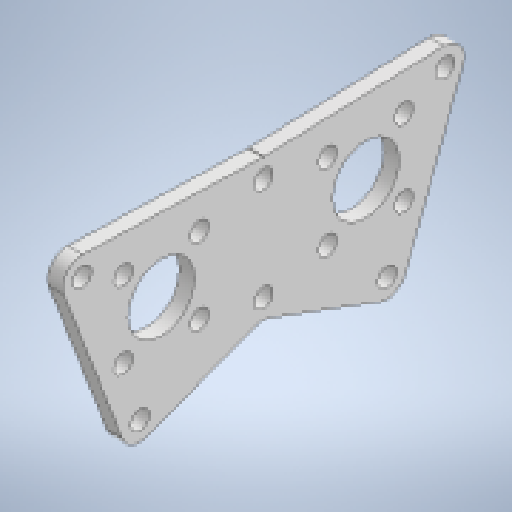
# Autodesk Inventor part: Motor Mount Plate
Saved by Autodesk Inventor 2023 (Build 270158000, 158)
## iProperties
Created: 2022-09-05
Part Number: Motor Mount Plate
Material: Generic
Document SubType Name: Modeling
Designer: deli
Density: 1 g/cm^3
Appearance: Default
Author: deli
Autodesk Inventor part; units mm, degrees
ref_plane "YZ Plane" through (0, 0, 0) normal (1, 0, 0) x (0, 1, 0)
ref_plane "XZ Plane" through (0, 0, 0) normal (0, 1, 0) x (-1, 0, 0)
ref_plane "XY Plane" through (0, 0, 0) normal (0, 0, 1) x (1, 0, 0)
sketch "Sketch1" plane through (0, 0, 0) normal (1, 0, 0) x (0, 1, 0)
  circle A0 centre (-80.8361, -46.4876) radius 7 projected
  circle A1 centre (-63.8866, -67.1825) radius 2 projected
  circle A2 centre (-97.7855, -67.1825) radius 2 projected
  circle A3 centre (-80.8361, -87.8774) radius 7 projected
  arc A4 (-59.8856, -67.0926) -> (-59.8856, -67.2723) centre (-55.8866, -67.1825) ccw
  arc A5 (-101.8421, -67.8529) -> (-101.8421, -66.512) centre (-105.7855, -67.1825) ccw
  arc A6 (-59.0871, -31.5608) -> (-63.7648, -27.5289) centre (-63.0861, -31.4709) ccw
  arc A7 (-103.2648, -34.3297) -> (-106.5295, -38.9422) centre (-102.5861, -38.2717) ccw
  arc A8 (-106.5295, -95.4227) -> (-103.2648, -100.0352) centre (-102.5861, -96.0932) ccw
  arc A9 (-63.7648, -106.836) -> (-59.0871, -102.8041) centre (-63.0861, -102.894) ccw
  circle A10 centre (-80.8361, -46.4876) radius 9.3137 construction
  circle A11 centre (-80.8361, -87.8774) radius 9.3137 construction
  circle A12 centre (-97.7855, -67.1825) radius 4 construction
  circle A13 centre (-63.8866, -67.1825) radius 4 construction
  line L0 (-63.7648, -27.5289) -> (-103.2648, -34.3297)
  line L1 (-106.5295, -38.9422) -> (-101.8421, -66.512)
  line L2 (-101.8421, -67.8529) -> (-106.5295, -95.4227)
  line L3 (-103.2648, -100.0352) -> (-63.7648, -106.836)
  line L4 (-59.8856, -67.0926) -> (-59.0871, -31.5608)
  line L5 (-59.8856, -67.2723) -> (-59.0871, -102.8041)
  circle A14 centre (-72.8361, -54.4876) radius 2
  circle A15 centre (-72.8361, -38.4876) radius 2
  circle A16 centre (-88.8361, -38.4876) radius 2
  circle A17 centre (-88.8361, -54.4876) radius 2
  circle A18 centre (-88.8361, -79.8774) radius 2
  circle A19 centre (-88.8361, -95.8774) radius 2
  circle A20 centre (-72.8361, -95.8774) radius 2
  circle A21 centre (-72.8361, -79.8774) radius 2
  line L6 (-72.8361, -38.4876) -> (-72.8361, -54.4876) construction
  line L7 (-72.8361, -54.4876) -> (-88.8361, -54.4876) construction
  line L8 (-88.8361, -54.4876) -> (-88.8361, -38.4876) construction
  line L9 (-88.8361, -38.4876) -> (-72.8361, -38.4876) construction
  line L10 (-72.8361, -79.8774) -> (-72.8361, -95.8774) construction
  line L11 (-72.8361, -95.8774) -> (-88.8361, -95.8774) construction
  line L12 (-88.8361, -95.8774) -> (-88.8361, -79.8774) construction
  line L13 (-88.8361, -79.8774) -> (-72.8361, -79.8774) construction
  circle A22 centre (-102.5861, -38.2717) radius 2 projected
  circle A23 centre (-63.0861, -31.4709) radius 2 projected
  circle A24 centre (-102.5861, -96.0932) radius 2 projected
  circle A25 centre (-63.0861, -102.894) radius 2 projected
  point P0 (0, 0)
  dimension "d31" = 8
  dimension "d32" = 8
  dimension "d33" = 8
  dimension "d34" = 8
  dimension "d35" = 8
  dimension "d36" = 8
  dimension "d37" = 8
  dimension "d38" = 8
  dimension "d39" = 0
  dimension "d40" = 0
  dimension "d41" = 4
  dimension "d42" = 4
  dimension "d43" = 4
  dimension "d44" = 4
  dimension "d45" = 4
  dimension "d46" = 4
  dimension "d47" = 4
  dimension "d48" = 4
  dimension "d49" = 16
  dimension "d50" = 16
  dimension "d51" = 16
  dimension "d52" = 16
  constraints: 28 end point, 22 tangent, 18 centre point, 12 point on circle, 4 coincident, 4 concentric, 4 perpendicular, 2 vertical
  measures "d31" diameter of A4
  measures "d32" diameter of A5
  measures "d33" diameter of A6
  measures "d34" diameter of A7
  measures "d35" diameter of A8
  measures "d36" diameter of A9
  measures "d37" diameter of A13
  measures "d38" diameter of A12
  measures "d39" vertical distance of A4.centre A1.centre
  measures "d40" vertical distance of A2.centre A5.centre
  measures "d41" diameter of A15
  measures "d42" diameter of A14
  measures "d43" diameter of A16
  measures "d44" diameter of A17
  measures "d45" diameter of A18
  measures "d46" diameter of A19
  measures "d47" diameter of A20
  measures "d48" diameter of A21
  measures "d49" distance of L6.start L6.end
  measures "d50" distance of L8.end L6.start
  measures "d51" distance of L10.start L10.end
  measures "d52" distance of L12.end L10.start
extrude "Extrusion1" add sketch "Sketch1" along normal blind 3.175 contours A4 L5 A9 L3 A8 L2 A5 L1 A7 L0 A6 L4 | A22 | A23 | A24 | A25
equation "\"d32\" = d31"
equation "\"d33\" = d31"
equation "\"d34\" = d31"
equation "\"d35\" = d31"
equation "\"d36\" = d31"
equation "\"d37\" = d31"
equation "\"d38\" = d37"
equation "\"d42\" = d41"
equation "\"d43\" = d41"
equation "\"d44\" = d41"
equation "\"d45\" = d41"
equation "\"d46\" = d41"
equation "\"d47\" = d41"
equation "\"d48\" = d41"
body "Solid1"
